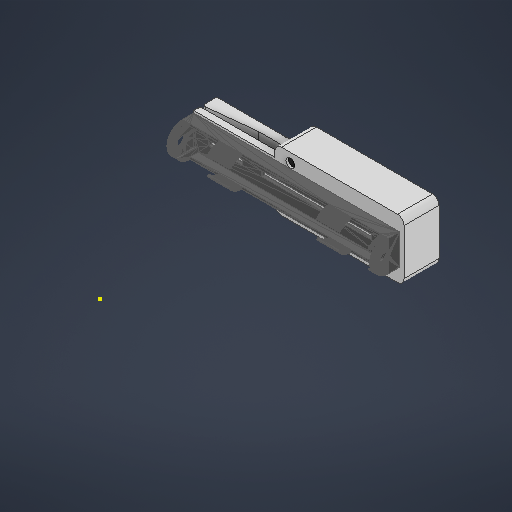
# Autodesk Inventor part: obj_1_电池盒.STEP
Saved by Autodesk Inventor 2025 (Build 290162000, 162)
## iProperties
Created: 2025-12-19
Part Number: obj_1_电池盒.STEP
Material: 常规
Document SubType Name: Modeling
Designer: XH
Density: 1 g/cm^3
Appearance: 默认
Author: XH
## iProperties of the stored document obj_1_电池盒.STEP_3D 打印.ipt
Created: 2025-12-20
Part Number: obj_1_电池盒.STEP_3D 打印
Material: 常规
Document SubType Name: Modeling
Designer: XH
Density: 1 g/cm^3
Appearance: 默认
Author: XH
Autodesk Inventor part; units mm, degrees
ref_plane "YZ Plane" through (0, 0, 0) normal (1, 0, 0) x (0, 1, 0)
ref_plane "XZ Plane" through (0, 0, 0) normal (0, 1, 0) x (-1, 0, 0)
ref_plane "XY Plane" through (0, 0, 0) normal (0, 0, 1) x (1, 0, 0)
sketch "草图1" plane through (42.95, 80.9918, 0) normal (0, 0, -1) x (-1, 0, 0)
  line L0 (-94.1, 15) -> (0, 15)
  line L1 (0, 15) -> (0, -1)
  line L2 (0, -1) -> (-94.1, -1)
  line L3 (-94.1, -1) -> (-94.1, 15)
  line L4 (0, 0) -> (0, 14) projected
  line L5 (-94.1, 14) -> (-94.1, 0) projected
  line L6 (0, 14) -> (-94.1, 14) projected
  line L7 (-94.1, 0) -> (0, 0) projected
  line L8 (-94.1, 7) -> (0, 7)
  line L9 (-39.1, -4.5) -> (-94.1, -4.5)
  line L10 (-94.1, -4.5) -> (-94.1, 18.5)
  line L11 (-94.1, 18.5) -> (-39.1, 18.5)
  line L12 (-39.1, 18.5) -> (-39.1, -4.5)
  line L13 (-39.1, -4.5) -> (-94.1, 18.5) construction
  line L14 (-94.1, -4.5) -> (-39.1, 18.5) construction
  point P0 (42.95, -80.9918)
  point P1 (-66.6, 7)
  point P2 (-39.1, -1)
  point P3 (-39.1, 15)
  dimension "d0" = 1
  dimension "d1" = 1
  dimension "d2" = 23
  dimension "d3" = 55
  constraints: 22 end point, 4 midpoint, 4 parallel, 3 collinear, 2 horizontal, 2 perpendicular, 1 point on line
  measures "d0" distance between parallel lines of L6 L0
  measures "d1" distance between parallel lines of L7 L2
  measures "d2" distance of L9.end L10.end
  measures "d3" distance between parallel lines of L12 L10
extrude "拉伸1" add sketch "草图1" along normal blind 1
sketch "草图2" plane through (42.95, 80.9918, -1) normal (0, 0, -1) x (-1, 0, 0)
  line L0 (-74.55, 0) -> (-74.55, -4.5) projected
  line L1 (-39.1, 18.5) -> (-94.1, 18.5) projected
  line L2 (-94.1, -4.5) -> (-39.1, -4.5)
  line L3 (-39.1, -4.5) -> (-39.1, 18.5)
  line L4 (-39.1, 18.5) -> (-94.1, 18.5)
  line L5 (-94.1, 18.5) -> (-94.1, -4.5)
  line L6 (-96.1, -6.5) -> (-37.1, -6.5)
  line L7 (-37.1, -6.5) -> (-37.1, 20.5)
  line L8 (-37.1, 20.5) -> (-96.1, 20.5)
  line L9 (-96.1, 20.5) -> (-96.1, -6.5)
  point P0 (42.95, -80.9918)
  dimension "d6" = 2
  constraints: 16 end point, 4 parallel, 2 perpendicular, 1 horizontal, 4 other
  measures "d6" distance between parallel lines of L5 L9
extrude "拉伸2" add sketch "草图2" against normal up to surface (1 mm away) contours L3 L2 L5 L1 | L9 L8 L7 L6
extrude "拉伸3" add sketch "草图2" along normal blind 15
fillet "圆角1" radius 2 1 edges at (80.05, 87.9918, -1)
sketch "草图3" plane through (42.95, 80.9918, 0) normal (0, 0, 1) x (1, 0, 0)
  point P0 (-42.95, -80.9918)
fillet "圆角2" radius 3 4 edges at (80.05, 74.4918, -8) (80.05, 101.4918, -8) (139.05, 74.4918, -8) (139.05, 101.4918, -8)
sketch "草图4" plane through (42.95, 79.9918, -1) normal (0, -1, 0) x (1, 0, 0)
  line L0 (0, 1) -> (0, 0) projected
  line L1 (37.1, 1) -> (37.1, -15) projected
  line L2 (0, 0) -> (37.1, 0)
  line L3 (37.1, 0) -> (37.1, -9.5558)
  line L4 (37.1, -9.5558) -> (0, -9.5558)
  line L5 (0, -9.5558) -> (0, 0)
  point P0 (-42.95, 1)
  point P1 (37.1, 0)
  constraints: 8 end point, 2 parallel, 1 horizontal, 1 perpendicular, 1 point on line
extrude "拉伸4" add sketch "草图4" against normal up to surface (16 mm away)
fillet "圆角3" radius 5.5 1 edges at (80.05, 87.9918, -10.5558)
sketch "草图5" plane through (42.95, 79.9918, 0) normal (0, -1, 0) x (1, 0, 0)
  line L0 (0, 0) -> (37.1, 0) projected
  line L1 (0, 0) -> (37.1, 0)
  line L2 (37.1, 0) -> (37.1, -3)
  line L3 (37.1, -3) -> (0, -3)
  line L4 (0, -3) -> (0, 0)
  line L5 (37.1, 0) -> (37.1, -16)
  line L6 (0, -3) -> (37.2428, -3)
  line L7 (37.2428, -3) -> (37.2428, -6.4975)
  line L8 (37.2428, -6.4975) -> (0, -6.4975)
  line L9 (0, -6.4975) -> (0, -3)
  line L10 (0, 0) -> (0, -10.5558) projected
  line L11 (0, -4) -> (23.3302, -6.4975)
  point P0 (-42.95, 0)
  point P1 (0, -4)
  point P2 (37.1, -7.9715)
  point P3 (37.1, -3)
  point P4 (37.1, -6.4975)
  dimension "d16" = 3
  dimension "d20" = 1
  constraints: 20 end point, 4 parallel, 2 horizontal, 2 perpendicular, 2 point on line
  measures "d16" distance between parallel lines of L0 L3
  measures "d20" distance of L3.end L11.start
extrude "拉伸5" cut sketch "草图5" against normal blind 61.75 contours L3 L5 L8 L11 L9
fillet "圆角4" radius 1 3 edges at (80.05, 87.9918, -3) (42.95, 87.9918, -4) (42.95, 87.9918, -3)
sketch "草图6" plane through (42.95, 80.9918, 0) normal (0, 0, 1) x (1, 0, 0)
  circle A0 centre (44.1719, 16.2818) radius 2
  point P0 (-42.95, -80.9918)
  dimension "d22" = 4
  constraints: 1 centre point
  measures "d22" diameter of A0
extrude "拉伸6" cut sketch "草图6" against normal blind 61.75
